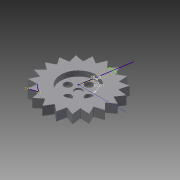
# Autodesk Inventor part: SmallGearV2
Saved by Autodesk Inventor 2015 (Build 190159000, 159)
## iProperties
Created: 2016-02-18
Part Number: SmallGearV2
Material: Generic
Document SubType Name: Modeling
Designer: Hatch
Density: 1 g/cm^3
Appearance: Default
Author: Hatch
Autodesk Inventor part; units mm, degrees
ref_plane "YZ Plane" through (0, 0, 0) normal (1, 0, 0) x (0, 1, 0)
ref_plane "XZ Plane" through (0, 0, 0) normal (0, 1, 0) x (-1, 0, 0)
ref_plane "XY Plane" through (0, 0, 0) normal (0, 0, 1) x (1, 0, 0)
sketch "Sketch1" plane through (0, 0, 0) normal (0, 1, 0) x (-1, 0, 0)
  circle A0 centre (0, 0) radius 16.6257
  dimension "d0" = 33.2513
  constraints: 1 centre point, 1 coincident
  measures "d0" diameter of A0
extrude "Extrusion1" add sketch "Sketch1" along normal blind 5
sketch "Sketch2" plane through (0, 5, 0) normal (0, 1, 0) x (1, 0, 0)
  circle A0 centre (0, 0) radius 10
  dimension "d3" = 20
  constraints: 1 centre point, 1 coincident
  measures "d3" diameter of A0
extrude "Extrusion2" cut sketch "Sketch2" against normal blind 3
sketch "Sketch3" plane through (0, 2, 0) normal (0, 1, 0) x (1, 0, 0)
  circle A0 centre (-6, 0) radius 2.125
  circle A1 centre (-6, 0) radius 2.125
  point P0 (0, 0)
  dimension "d7" = 4.25
  constraints: 2 centre point, 1 coincident, 1 concentric
  measures "d7" diameter of A0
extrude "Extrusion3" cut sketch "Sketch3" against normal through all
pattern_circular "Circular Pattern1" count 4 over 360 about axis through (0, 5, 0) along (0, -1, 0) of "Extrusion3"
sketch "Sketch4" plane through (0, 2, 0) normal (0, 1, 0) x (1, 0, 0)
  circle A0 centre (0, 0) radius 2.125
  dimension "d13" = 4.25
  constraints: 1 centre point, 1 coincident
  measures "d13" diameter of A0
extrude "Extrusion4" cut sketch "Sketch4" against normal blind 1
sketch "Sketch6" plane through (0, 5, 0) normal (0, 1, 0) x (1, 0, 0)
  arc A0 (5.4078, 16.6435) -> (0, 17.5) centre (0, 0) ccw
  line L0 (0, 0) -> (5.4078, 16.6435) construction
  line L1 (0, 0) -> (0, 17.5) construction
  line L2 (0, 0) -> (4.3015, 27.1585)
  line L3 (0, 0) -> (27.497, 0) construction
  arc A1 (5.4078, 16.6435) -> (0, 17.5) centre (0, 0) ccw
  dimension "d16" = 18
  dimension "d17" = 81
  constraints: 8 end point, 4 point on circle, 2 centre point, 1 coincident, 1 equal length, 1 horizontal
  measures "d16" angle of L0 L1
  measures "d17" angle of L3 L2
sketch "Sketch7" plane through (0, 5, 0) normal (0, 1, 0) x (1, 0, 0)
  circle A0 centre (0, 0) radius 16.6257 projected
  arc A1 (5.1376, 15.8119) -> (0, 16.6257) centre (0, 0) ccw
  line L0 (0, 0) -> (5.1376, 15.8119) construction
  line L1 (0, 0) -> (0, 16.6257) construction
  line L2 (0, 0) -> (4.2807, 27.027)
  line L3 (0, 0) -> (27.3639, 0) construction
  line L4 (0, 16.6257) -> (3.2368, 20.4365)
  line L5 (3.2368, 20.4365) -> (5.1376, 15.8119)
  dimension "d18" = 18
  dimension "d19" = 81
  dimension "d20" = 5
  constraints: 12 end point, 2 point on circle, 1 centre point, 1 coincident, 1 equal length, 1 horizontal, 1 point on line, 1 vertical alignment, 1 other
  measures "d18" angle of L0 L1
  measures "d19" angle of L3 L2
  measures "d20" distance of L1.end L4.end
extrude "Extrusion5" add sketch "Sketch7" against normal blind 5 contours A0 L2 L5 | L4 L2 A0
pattern_circular "Circular Pattern2" count 19 over 360 about axis through (0, 0, 0) along (0, 1, 0) of "Extrusion5"
sketch "Sketch8" plane through (0, 5, 0) normal (0, 1, 0) x (1, 0, 0)
  point P0 (0, 0)
sketch "Sketch9" plane through (0, 5, 0) normal (0, 1, 0) x (1, 0, 0)
  arc A0 (-12.044, -11.4609) -> (-7.9129, -14.6218) centre (0, 0) ccw
  line L0 (-7.9129, -14.6218) -> (-12.5734, -16.4328)
  line L1 (-7.9129, -14.6218) -> (-12.5734, -16.4328) projected
  constraints: 2 end point, 2 point on circle, 1 centre point, 1 coincident, 1 collinear
body "Solid1"
